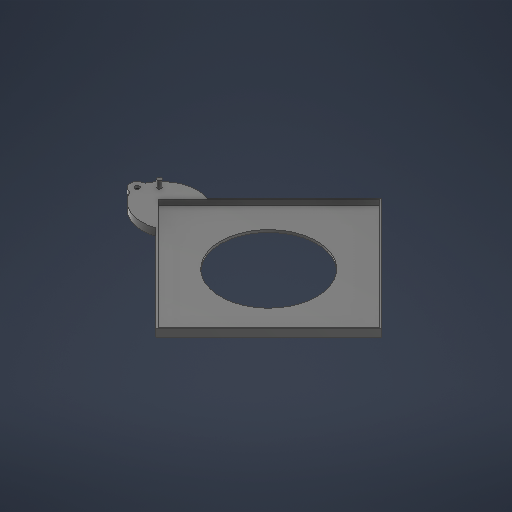
# Autodesk Inventor part: flowerstand
Saved by Autodesk Inventor 2027 (Build 310192060, 192F)
## iProperties
Created: 2026-05-29
Part Number: flowerstand
Material: Ogólny
Document SubType Name: Modeling
Designer: User
Density: 1 g/cm^3
Appearance: Domyślna
Author: User
Autodesk Inventor part; units mm, degrees
ref_plane "YZ Plane" through (0, 0, 0) normal (1, 0, 0) x (0, 1, 0)
ref_plane "XZ Plane" through (0, 0, 0) normal (0, 1, 0) x (-1, 0, 0)
ref_plane "XY Plane" through (0, 0, 0) normal (0, 0, 1) x (1, 0, 0)
sketch "Szkic4" plane through (0, 0, 0) normal (0, 1, 0) x (-1, 0, 0)
  circle A0 centre (0, 0) radius 2.1
  line L0 (-3, 3) -> (3, 3)
  line L1 (3, 3) -> (3, -3)
  line L2 (3, -3) -> (-3, -3)
  line L3 (-3, -3) -> (-3, 3)
  line L4 (-3, 3) -> (3, -3) construction
  line L5 (3, 3) -> (-3, -3) construction
  line L6 (0, 0) -> (-4.5962, -4.5962)
  line L7 (0, 0) -> (6.5, 0) construction
  line L8 (0, 0) -> (-4.5962, 4.5962)
  line L9 (0, 0) -> (6.5, 0) construction
  arc A1 (-4.5962, 4.5962) -> (-4.5962, -4.5962) centre (0, 0) ccw construction
  arc A2 (-5.3033, 5.3033) -> (-5.3033, -5.3033) centre (0, 0) ccw
  arc A3 (-3.8891, 3.8891) -> (-3.8891, -3.8891) centre (0, 0) ccw
  arc A4 (-3.8891, 3.8891) -> (-5.3033, 5.3033) centre (-4.5962, 4.5962) ccw
  arc A5 (-5.3033, -5.3033) -> (-3.8891, -3.8891) centre (-4.5962, -4.5962) ccw
  line L10 (0, 0) -> (-7.7, 0)
  line L11 (0, 0) -> (7.7, 0) construction
  line L12 (-7.7, 0) -> (-54.7226, -47.0226)
  line L13 (-54.7226, -47.0226) -> (-101.7452, 0)
  line L14 (-101.7452, 0) -> (-54.7226, 47.0226)
  line L15 (-54.7226, 47.0226) -> (-7.7, 0)
  line L16 (-7.7, 0) -> (58.8, 0) construction
  line L17 (-7.7, 0) -> (-8.7, 0)
  line L18 (-8.7, 0) -> (-54.6619, -45.9619)
  line L19 (-54.6619, -45.9619) -> (-100.6239, 0)
  line L20 (-100.6239, 0) -> (-54.6619, 45.9619)
  line L21 (-54.6619, 45.9619) -> (-8.7, 0)
  line L22 (-8.7, 0) -> (56.3, 0) construction
  arc A6 (-18.4411, -10.7411) -> (0, -3) centre (-13.548, 3.4383) ccw
  arc A7 (0, 3) -> (-18.4411, 10.7411) centre (-13.548, -3.4383) ccw
  point P0 (-18.4411, 10.7411)
  point P1 (0, 3)
  point P2 (-3, 0)
  dimension "d52" = 4.2
  dimension "d53" = 6
  dimension "d54" = 6
  dimension "d55" = 6.5
  dimension "d56" = 135
  dimension "d57" = 6.5
  dimension "d58" = 135
  dimension "d59" = 6.5
  dimension "d60" = 2
  dimension "d61" = 7.7
  dimension "d62" = 180
  dimension "d67" = 66.5
  dimension "d68" = 135
  dimension "d69" = 66.5
  dimension "d70" = 1
  dimension "d71" = 65
  dimension "d72" = 135
  dimension "d73" = 65
  dimension "d74" = 20
  dimension "d75" = 15
  constraints: 46 end point, 14 point on circle, 8 centre point, 8 horizontal, 7 parallel, 5 equal length, 4 midpoint, 4 tangent, 3 perpendicular, 3 symmetric about line, 2 collinear, 1 coincident, 1 point on line, 1 other
  measures "d52" diameter of A0
  measures "d53" distance of L1.end L2.end
  measures "d54" distance of L0.end L1.end
  measures "d55" distance of L6.start L6.end
  measures "d56" angle of L6 L7
  measures "d57" distance of L6.start L8.end
  measures "d58" angle of L9 L8
  measures "d59" radius of A1
  measures "d60" diameter of A5
  measures "d61" distance of L10.start L10.end
  measures "d62" angle of L10 L11
  measures "d67" distance of L10.end L12.end
  measures "d68" angle of L12 L16
  measures "d69" distance of L12.end L13.end
  measures "d70" distance of L10.end L17.end
  measures "d71" distance of L17.end L18.end
  measures "d72" angle of L18 L22
  measures "d73" distance of L18.end L19.end
  measures "d74" distance of A6.end A6.start
  measures "d75" radius of A6
extrude "Wyciągnięcie proste4" add sketch "Szkic4" along normal blind 3 contours A0 L8 L0 L1 L2 L6 | A0 L10 L3 L8 | L6 L3 L10 A0 | L8 A4 A2 L10 L15 A7 L0 | L3 L10 A3 L8 | L6 A3 L10 L3 | L2 A6 L12 L10 A2 A5 L6 | L15 L12 L13 L14
extrude "Wyciągnięcie proste5" add sketch "Szkic4" along normal blind 1 contours L18 L19 L20 L21
surface extrude "PowWyciągnięciaProstego2" sketch "Szkic4" along normal blind 5.5 shown no curves A3 A4 A2 A5
fillet "Zaokrąglenie1" radius 3 2 edges at (-3, 1.5, 3) (-3, 1.5, -3)
sketch "Szkic5" plane through (0, 1, 0) normal (0, 1, 0) x (1, 0, 0)
  line L0 (8.7, 0) -> (54.6619, 45.9619) projected
  line L1 (8.7, 0) -> (100.6239, 0)
  circle A0 centre (54.6619, 0) radius 20
  point P0 (0, 0)
  dimension "d84" = 40
  constraints: 2 end point, 1 centre point, 1 midpoint
  measures "d84" diameter of A0
extrude "Wyciągnięcie proste6" cut sketch "Szkic5" against normal blind 10
sketch "Szkic6" plane through (0, 3, 0) normal (0, 1, 0) x (1, 0, 0)
  arc A0 (3.8891, -3.8891) -> (3.8891, 3.8891) centre (0, 0) ccw projected
  arc A1 (3.8891, -3.8891) -> (5.3033, -5.3033) centre (4.5962, -4.5962) ccw projected
  arc A2 (5.3033, -5.3033) -> (5.3033, 5.3033) centre (0, 0) ccw projected
  arc A3 (5.3033, 5.3033) -> (3.8891, 3.8891) centre (4.5962, 4.5962) ccw projected
  line L0 (0, 0) -> (4.5962, 4.5962)
  circle A4 centre (4.5962, 4.5962) radius 0.9
  circle A5 centre (0, 0) radius 2.1
  circle A6 centre (0, 0) radius 1
  point P0 (0, 0)
  dimension "d87" = 1.8
  dimension "d92" = 2
  constraints: 3 centre point, 3 coincident, 2 end point
  measures "d87" diameter of A4
  measures "d92" diameter of A6
extrude "Wyciągnięcie proste7" add sketch "Szkic6" against normal blind 1 contours A0 A3 A2 A1 | A4 | A5
extrude "Wyciągnięcie proste8" add sketch "Szkic6" along normal blind 3 contours A4
body "Srf3"
